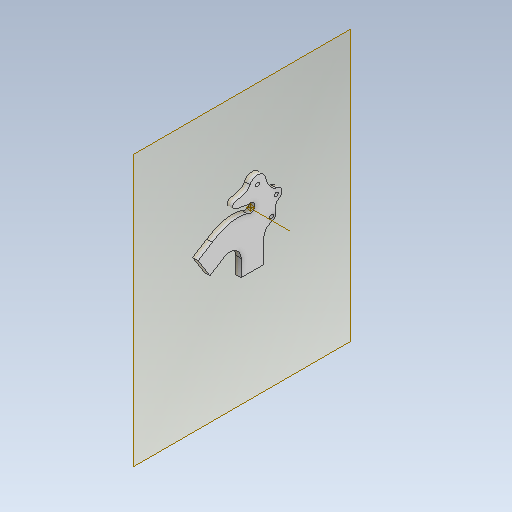
# Autodesk Inventor part: soporte_eje_trasero
Saved by Autodesk Inventor 2021 (Build 250183000, 183)
## iProperties
Created: 2021-04-09
Part Number: soporte_eje_trasero
Material: Genérico
Document SubType Name: Modeling
Designer: j2seb
Density: 1 g/cm^3
Appearance: Valor por defecto
Author: j2seb
Autodesk Inventor part; units mm, degrees
ref_plane "YZ Plane" through (0, 0, 0) normal (1, 0, 0) x (0, 1, 0)
ref_plane "XZ Plane" through (0, 0, 0) normal (0, 1, 0) x (-1, 0, 0)
ref_plane "XY Plane" through (0, 0, 0) normal (0, 0, 1) x (1, 0, 0)
ref_plane "Plano de trabajo1" through (-185.7873, -389.4877, 168.7004) normal (1, 0, 0) x (0, 1, 0)
sketch "Boceto1" plane through (-185.7873, -389.4877, 168.7004) normal (1, 0, 0) x (0, 1, 0)
  spline S0 degree 3 poles (534.733, 23.2998) (534.7105, 23.7942) (534.6906, 24.2218) (534.6565, 24.9274) (534.6425, 25.2033) (534.6129, 25.7399) (534.6044, 25.8219) (534.6094, 25.4554) (534.6229, 25.0104) (534.6701, 23.6469) (534.7034, 22.7415) (534.7857, 20.5852) (534.8338, 19.3549) (534.9389, 16.7287) (534.9948, 15.3579) (535.1069, 12.6551) (535.1621, 11.3489) (535.2644, 8.9741) (535.3106, 7.9282) (535.3879, 6.2371) (535.4183, 5.608) (535.4589, 4.8538) (535.4688, 4.7358) (535.4667, 5.0314) (535.4548, 5.4422) (535.4103, 6.7433) (535.3782, 7.6213) (535.2979, 9.7332) (535.2505, 10.9469) (535.1465, 13.5533) (535.0909, 14.9211) (534.9787, 17.6317) (534.9233, 18.9486) (534.8197, 21.3576) (534.7727, 22.4265) (534.733, 23.2998) knots -6.594944 -6.594944 -6.594944 -6.594944 -6.363484 -6.363484 -6.132024 -6.132024 -5.723223 -5.723223 -5.314421 -5.314421 -4.90562 -4.90562 -4.496818 -4.496818 -4.088016 -4.088016 -3.679215 -3.679215 -3.270413 -3.270413 -2.861611 -2.861611 -2.45281 -2.45281 -2.044008 -2.044008 -1.635207 -1.635207 -1.226405 -1.226405 -0.817603 -0.817603 -0.408802 -0.408802 0 0 0 0 construction
  spline S1 degree 3 poles (563.9582, 57.2503) (564.369, 57.506) (564.6982, 57.7109) (565.1814, 58.0114) (565.334, 58.1062) (565.502, 58.21) (565.3211, 58.0968) (564.4035, 57.5239) (563.6756, 57.0698) (561.7633, 55.8774) (560.5973, 55.1504) (557.9767, 53.5169) (556.5472, 52.6259) (553.6106, 50.7959) (552.1317, 49.8744) (549.319, 48.122) (548.0121, 47.3078) (545.7443, 45.8954) (544.8051, 45.3106) (543.4219, 44.4496) (542.9911, 44.1816) (542.6995, 44.001) (542.8416, 44.0901) (543.6854, 44.617) (544.379, 45.0497) (546.2318, 46.2051) (547.3731, 46.9167) (549.9574, 48.5276) (551.3756, 49.4116) (554.3045, 51.2368) (555.7872, 52.1607) (558.622, 53.9269) (559.9471, 54.7524) (562.2635, 56.1952) (563.2327, 56.7987) (563.9582, 57.2503) knots -8.403752 -8.403752 -8.403752 -8.403752 -8.108809 -8.108809 -7.813866 -7.813866 -7.292942 -7.292942 -6.772017 -6.772017 -6.251093 -6.251093 -5.730168 -5.730168 -5.209244 -5.209244 -4.68832 -4.68832 -4.167395 -4.167395 -3.646471 -3.646471 -3.125546 -3.125546 -2.604622 -2.604622 -2.083698 -2.083698 -1.562773 -1.562773 -1.041849 -1.041849 -0.520924 -0.520924 0 0 0 0 construction
  spline S2 degree 3 poles (534.6356, 25.8056) (534.6632, 25.2036) (534.6939, 24.5175) (534.7607, 23.0024) (534.7966, 22.178) (534.9005, 19.7543) (534.9715, 18.0684) (535.1144, 14.6095) (535.185, 12.8696) (535.3167, 9.5648) (535.3764, 8.0315) (535.4771, 5.3755) (535.517, 4.2783) (535.5717, 2.669) (535.5858, 2.1723) (535.5862, 1.8506) (535.5724, 2.0287) (535.5185, 3.0427) (535.4789, 3.869) (535.3787, 6.0669) (535.3192, 7.4176) (535.1878, 10.4704) (535.1173, 12.1433) (534.9744, 15.5937) (534.9034, 17.3383) (534.7703, 20.6697) (534.7095, 22.2248) (534.6062, 24.9384) (534.5647, 26.071) (534.5067, 27.7605) (534.4907, 28.3011) (534.4865, 28.7134) (534.4984, 28.5811) (534.5489, 27.6545) (534.5869, 26.869) (534.6356, 25.8056) knots -8.403752 -8.403752 -8.403752 -8.403752 -8.108809 -8.108809 -7.813866 -7.813866 -7.292942 -7.292942 -6.772017 -6.772017 -6.251093 -6.251093 -5.730168 -5.730168 -5.209244 -5.209244 -4.68832 -4.68832 -4.167395 -4.167395 -3.646471 -3.646471 -3.125546 -3.125546 -2.604622 -2.604622 -2.083698 -2.083698 -1.562773 -1.562773 -1.041849 -1.041849 -0.520924 -0.520924 0 0 0 0 construction
  line L0 (525, 5.254) -> (525, 25.254)
  line L1 (525, 25.254) -> (540, 25.254)
  arc A0 (540, 25.254) -> (548.4852, 40.5618) centre (540, 35.2596) ccw
  line L2 (548.4852, 40.5618) -> (540.5364, 53.2825)
  line L3 (540.5364, 53.2825) -> (557.4974, 63.8809)
  line L4 (557.4974, 63.8809) -> (565.4462, 51.1602)
  line L5 (525, 15.254) -> (575, 17.0001) construction
  line L6 (549.0169, 58.5817) -> (575, 17.0001) construction
  line L7 (525, 5.254) -> (540, 5.254)
  circle A1 centre (575, 17.0001) radius 4 construction
  line L8 (565.4462, 51.1602) -> (573.2852, 38.6152) construction
  line L9 (573.8755, 23.7788) -> (571.0024, 16.8605) construction
  spline S3 degree 4 poles (565.4462, 51.1602) (573.2852, 38.6152) (573.8755, 31.3158) (573.8755, 23.7788) (571.0024, 16.8605) knots 1 1 1 1 1 2 2 2 2 2
  circle A2 centre (575, 17.0001) radius 4
  line L10 (578.9765, 17.4327) -> (578.7688, 19.3424) construction
  line L11 (578.7688, 19.3424) -> (580.8115, 30.4088) construction
  line L12 (580.8115, 30.4088) -> (581.5561, 33.9943) construction
  line L13 (581.5561, 33.9943) -> (588.3082, 32.4831) construction
  line L14 (588.3082, 32.4831) -> (587.0334, 24.49) construction
  line L15 (587.0334, 24.49) -> (590.1956, 18.7656) construction
  line L16 (546.3222, 5.254) -> (540, 5.254) construction
  line L17 (573.2852, 38.6152) -> (573.8755, 31.3158) construction
  line L18 (573.8755, 31.3158) -> (573.8755, 23.7788) construction
  arc A3 (591.5375, 3.1103) -> (593.375, 17.2458) centre (590.1405, 10.4791) ccw
  arc A4 (569.6718, -8.8556) -> (579.02, -6.402) centre (574.02, -6.3872) ccw
  arc A5 (555.1918, -3.2238) -> (560.0425, -5.8618) centre (559, -2) ccw
  spline S4 degree 4 poles (578.9765, 17.4327) (578.7688, 19.3424) (580.8115, 30.4088) (581.5561, 33.9943) (588.3082, 32.4831) (587.0334, 24.49) (590.1956, 18.7656) (593.375, 17.2458) knots 0 0 0 0 0 1 2 3 4 4 4 4 4
  line L19 (590.1956, 18.7656) -> (593.375, 17.2458) construction
  spline S5 degree 4 poles (555.1918, -3.2238) (553.3097, 2.6327) (551.1077, 4.616) (546.3222, 5.254) (540, 5.254) knots 21.570729 21.570729 21.570729 21.570729 21.570729 22 22 22 22 22
  line L20 (555.1918, -3.2238) -> (553.3097, 2.6327) construction
  line L21 (553.3097, 2.6327) -> (551.1077, 4.616) construction
  line L22 (551.1077, 4.616) -> (546.3222, 5.254) construction
  line L23 (569.6718, -8.8556) -> (566.9184, -4.0055) construction
  line L24 (566.9184, -4.0055) -> (560.0425, -5.8618) construction
  spline S6 degree 2 poles (569.6718, -8.8556) (566.9184, -4.0055) (560.0425, -5.8618) knots 1 1 1 2 2 2
  line L25 (575, 17.0001) -> (528.8996, 17.0001) construction
  line L26 (591.5375, 3.1103) -> (584.136, 1.7072) construction
  line L27 (584.136, 1.7072) -> (579.0273, -3.9321) construction
  line L28 (579.0273, -3.9321) -> (579.02, -6.402) construction
  spline S7 degree 3 poles (591.5375, 3.1103) (584.136, 1.7072) (579.0273, -3.9321) (579.02, -6.402) knots 1 1 1 1 2 2 2 2
  point P0 (389.4877, -168.7004)
  point P1 (534.733, 23.2998)
  point P2 (563.9582, 57.2503)
  point P3 (534.6356, 25.8056)
  point P4 (571.974, 19.6161)
  point P5 (578.9765, 17.4332)
  point P6 (571.0024, 16.8605)
  dimension "d78" = 8
  dimension "d75" = 20
  dimension "d76" = 60
  dimension "d77" = 15
  dimension "d232" = 15
  dimension "d233" = 10
  dimension "d234" = 8
  dimension "d290" = 2
  dimension "d291" = 50
  constraints: 18 end point, 8 point on circle, 4 centre point, 4 coincident, 4 equal length, 3 horizontal, 2 midpoint, 2 parallel, 2 perpendicular, 2 tangent, 1 point on line, 1 vertical, 29 other
  measures "d75" distance of L0.start L0.end
  measures "d76" angle of L5 L6
  measures "d77" distance of L0.start L7.end
  measures "d232" diameter of A3
  measures "d233" diameter of A4
  measures "d234" diameter of A5
  measures "d290" angle of L5 L25
  measures "d291" distance from line of L0 point (575, 17)
extrude "Extrusión1" add sketch "Boceto1" along normal mid plane 5 contours L0 L1 A0 L2 L3 L4 S3 A2 S4 A3 S7 A4 S6 A5 S5 L7
sketch "Boceto2" plane through (-188.2873, -389.4877, 168.7004) normal (-1, 0, 0) x (0, 0, 1)
  arc A0 (-5.8618, 560.0425) -> (-3.2238, 555.1918) centre (-2, 559) ccw projected
  arc A1 (-6.402, 579.02) -> (-8.8556, 569.6718) centre (-6.3872, 574.02) ccw projected
  arc A2 (17.2458, 593.375) -> (3.1103, 591.5375) centre (10.4791, 590.1405) ccw projected
  point P0 (-168.7004, 389.4877)
  constraints: 3 coincident
hole "Agujero1" at (-188.2873, 169.5123, 166.7004) at (-188.2873, 184.5323, 162.3132) at (-188.2873, 200.6529, 179.1795) direction (1, 0, 0) diameter 3.4 end through all clearance for "Tornillo para maquinaria de cabeza plana" size "M3" standard "Perfil M métrico ANSI"
